Autodesk Fusion 360 part; units mm, degrees
(part 16 of 25)
  arc A4090 (51.0803, 16.2122) -> (51.2018, 15.9188) centre (51.1411, 16.0655) ccw
  arc A4091 (50.459, 16.2243) -> (50.459, 15.9068) centre (50.459, 16.0655) ccw
  arc A4092 (53.8327, 16.4318) -> (54.0572, 16.2072) centre (53.9449, 16.3195) ccw
  arc A4093 (54.9592, 17.78) -> (54.6417, 17.78) centre (54.8005, 17.78) ccw
  arc A4094 (54.9128, 17.0628) -> (54.6882, 17.2873) centre (54.8005, 17.175) ccw
  arc A4095 (49.2443, 18.121) -> (48.9268, 18.121) centre (49.0856, 18.121) ccw
  arc A4096 (49.2343, 18.8634) -> (49.4588, 18.6389) centre (49.3465, 18.7512) ccw
  arc A4097 (53.34, 16.1608) -> (53.34, 16.4783) centre (53.34, 16.3195) ccw
  arc A4098 (52.3619, 16.6927) -> (52.1374, 16.9172) centre (52.2497, 16.805) ccw
  line L1395 (49.3465, 18.7512) -> (49.0855, 18.121)
  arc A4099 (53.34, 17.9387) -> (53.34, 17.6212) centre (53.34, 17.78) ccw
  line L1396 (52.735, 16.3195) -> (53.34, 16.3195)
  arc A4100 (49.8896, 16.4732) -> (49.7681, 16.1798) centre (49.8289, 16.3265) ccw
  arc A4101 (53.1812, 16.3195) -> (53.4987, 16.3195) centre (53.34, 16.3195) ccw
  arc A4102 (51.8319, 16.1798) -> (51.7104, 16.4732) centre (51.7712, 16.3265) ccw
  arc A4103 (53.4988, 17.78) -> (53.1813, 17.78) centre (53.3401, 17.78) ccw
  line L1397 (53.34, 16.3195) -> (53.34, 17.78)
  line L1398 (49.8288, 16.3265) -> (50.459, 16.0655)
  line L1399 (50.459, 16.0655) -> (51.141, 16.0655)
  line L1400 (49.0855, 17.439) -> (49.3465, 16.8088)
  arc A4104 (52.735, 16.4783) -> (52.735, 16.1608) centre (52.735, 16.3195) ccw
  line L1401 (49.0855, 18.121) -> (49.0855, 17.439)
  arc A4105 (50.3982, 15.9188) -> (50.5197, 16.2122) centre (50.459, 16.0655) ccw
  arc A4106 (54.8005, 17.6212) -> (54.8005, 17.9387) centre (54.8005, 17.78) ccw
  arc A4107 (53.34, 17.6212) -> (53.34, 17.9387) centre (53.34, 17.78) ccw
  arc A4108 (49.7166, 16.2143) -> (49.9411, 16.4388) centre (49.8288, 16.3266) ccw
  arc A4109 (49.2322, 17.4997) -> (48.9388, 17.3782) centre (49.0855, 17.439) ccw
  arc A4110 (49.4588, 16.9211) -> (49.2343, 16.6966) centre (49.3465, 16.8089) ccw
  arc A4111 (53.4988, 17.78) -> (53.1813, 17.78) centre (53.3401, 17.78) ccw
  arc A4112 (73.8187, 45.72) -> (73.5012, 45.72) centre (73.66, 45.72) ccw
  line L1402 (49.53, 40.64) -> (50.8, 41.91)
  arc A4113 (13.8113, 33.909) -> (14.1288, 33.909) centre (13.9701, 33.909) ccw
  arc A4114 (21.59, 12.5413) -> (21.59, 12.8588) centre (21.59, 12.7001) ccw
  line L1403 (33.02, 6.35) -> (35.56, 6.35)
  arc A4115 (15.1531, 11.5296) -> (15.3777, 11.305) centre (15.2654, 11.4173) ccw
  arc A4116 (72.5023, 47.1023) -> (72.2777, 46.8777) centre (72.39, 46.99) ccw
  arc A4117 (35.56, 6.1913) -> (35.56, 6.5088) centre (35.56, 6.3501) ccw
  arc A4118 (80.7491, 2.7242) -> (80.7491, 3.0417) centre (80.7491, 2.883) ccw
  arc A4119 (73.8187, 44.45) -> (73.5012, 44.45) centre (73.66, 44.45) ccw
  line L1404 (80.7212, 16.7894) -> (74.2188, 16.7894)
  arc A4120 (16.5481, 12.8588) -> (16.5481, 12.5413) centre (16.5481, 12.7001) ccw
  arc A4121 (3.1603, 40.2443) -> (2.9357, 40.0197) centre (3.048, 40.132) ccw
  line L1405 (80.7491, 2.8829) -> (74.2467, 2.8829)
  line L1406 (21.59, 12.7) -> (22.86, 13.97)
  arc A4122 (13.8577, 35.4477) -> (14.0823, 35.6723) centre (13.97, 35.56) ccw
  line L1407 (3.048, 41.91) -> (3.048, 40.132)
  arc A4123 (14.1288, 35.56) -> (13.8113, 35.56) centre (13.9701, 35.56) ccw
  arc A4124 (72.2313, 46.99) -> (72.5487, 46.99) centre (72.39, 46.99) ccw
  arc A4125 (80.7212, 16.6306) -> (80.7212, 16.9482) centre (80.7212, 16.7894) ccw
  line L1408 (50.8, 41.91) -> (52.07, 43.18)
  arc A4126 (11.43, 37.9413) -> (11.43, 38.2587) centre (11.43, 38.1) ccw
  arc A4127 (43.2923, 40.5277) -> (43.0677, 40.7523) centre (43.18, 40.64) ccw
  arc A4128 (50.6877, 42.0223) -> (50.9123, 41.7977) centre (50.8, 41.91) ccw
  line L1409 (13.97, 35.56) -> (13.97, 33.909)
  arc A4129 (33.02, 6.5088) -> (33.02, 6.1913) centre (33.02, 6.3501) ccw
  arc A4130 (73.5477, 45.6077) -> (73.7723, 45.8323) centre (73.66, 45.72) ccw
  line L1410 (3.048, 40.132) -> (5.08, 38.1)
  arc A4131 (74.2467, 3.0417) -> (74.2467, 2.7242) centre (74.2467, 2.883) ccw
  line L1411 (52.07, 43.18) -> (58.42, 43.18)
  line L1412 (43.18, 40.64) -> (49.53, 40.64)
  arc A4132 (21.4777, 12.8123) -> (21.7023, 12.5877) centre (21.59, 12.7) ccw
  arc A4133 (74.2188, 16.6306) -> (74.2188, 16.9482) centre (74.2188, 16.7894) ccw
  arc A4134 (50.6877, 29.0977) -> (50.9123, 29.3223) centre (50.8, 29.21) ccw
  arc A4135 (5.08, 38.2587) -> (5.08, 37.9413) centre (5.08, 38.1) ccw
  line L1413 (16.5481, 12.7) -> (21.59, 12.7)
  arc A4136 (73.5012, 31.75) -> (73.8187, 31.75) centre (73.66, 31.75) ccw
  arc A4137 (74.2188, 16.9482) -> (74.2188, 16.6306) centre (74.2188, 16.7894) ccw
  arc A4138 (2.8893, 40.132) -> (3.2067, 40.132) centre (3.048, 40.132) ccw
  line L1414 (73.66, 45.72) -> (72.39, 46.99)
  arc A4139 (68.4213, 19.05) -> (68.7387, 19.05) centre (68.58, 19.05) ccw
  arc A4140 (16.6604, 12.5877) -> (16.4358, 12.8123) centre (16.5481, 12.7) ccw
  arc A4141 (50.9588, 29.21) -> (50.6413, 29.21) centre (50.8001, 29.21) ccw
  line L1415 (15.2654, 11.4173) -> (16.5481, 12.7)
  arc A4142 (3.2067, 41.91) -> (2.8893, 41.91) centre (3.048, 41.91) ccw
  arc A4143 (49.53, 40.4813) -> (49.53, 40.7987) centre (49.53, 40.64) ccw
  arc A4144 (40.5277, 38.2123) -> (40.7523, 37.9877) centre (40.64, 38.1) ccw
  line L1416 (22.86, 13.97) -> (22.86, 16.51)
  arc A4145 (43.18, 40.7987) -> (43.18, 40.4813) centre (43.18, 40.64) ccw
  arc A4146 (22.7012, 13.97) -> (23.0188, 13.97) centre (22.86, 13.97) ccw
  line L1417 (40.64, 33.02) -> (46.99, 33.02)
  arc A4147 (47.1023, 33.1323) -> (46.8777, 32.9077) centre (46.99, 33.02) ccw
  line L1418 (73.66, 44.45) -> (73.66, 45.72)
  line L1419 (5.08, 38.1) -> (11.43, 38.1)
  line L1420 (73.66, 31.75) -> (73.66, 44.45)
  arc A4148 (11.5423, 38.2123) -> (11.3177, 37.9877) centre (11.43, 38.1) ccw
  line L1421 (11.43, 38.1) -> (13.97, 35.56)
  line L1422 (72.39, 46.99) -> (72.39, 49.53)
  arc A4149 (4.9677, 37.9877) -> (5.1923, 38.2123) centre (5.08, 38.1) ccw
  arc A4150 (23.0188, 16.51) -> (22.7012, 16.51) centre (22.86, 16.51) ccw
  arc A4151 (22.9723, 13.8577) -> (22.7477, 14.0823) centre (22.86, 13.97) ccw
  arc A4152 (73.5012, 44.45) -> (73.8187, 44.45) centre (73.66, 44.45) ccw
  arc A4153 (72.5487, 49.53) -> (72.2313, 49.53) centre (72.39, 49.53) ccw
  arc A4154 (16.002, 26.0668) -> (16.002, 25.7492) centre (16.002, 25.908) ccw
  arc A4155 (73.5012, 29.21) -> (73.8187, 29.21) centre (73.66, 29.21) ccw
  line L1423 (63.5, 31.75) -> (63.5, 29.21)
  arc A4156 (40.64, 33.1788) -> (40.64, 32.8613) centre (40.64, 33.0201) ccw
  line L1424 (68.58, 20.32) -> (70.485, 22.225)
  arc A4157 (26.5113, 25.4) -> (26.8288, 25.4) centre (26.67, 25.4) ccw
  line L1425 (68.58, 19.05) -> (68.58, 20.32)
  line L1426 (26.67, 29.21) -> (26.67, 25.4)
  arc A4158 (58.42, 43.0213) -> (58.42, 43.3387) centre (58.42, 43.18) ccw
  line L1427 (46.99, 33.02) -> (50.8, 29.21)
  line L1428 (33.02, 6.35) -> (30.48, 6.35)
  arc A4159 (26.67, 25.2413) -> (26.67, 25.5588) centre (26.67, 25.4001) ccw
  arc A4160 (73.7723, 29.0977) -> (73.5477, 29.3223) centre (73.66, 29.21) ccw
  line L1429 (73.66, 29.21) -> (73.66, 31.75)
  line L1430 (50.8, 29.21) -> (50.8, 25.4)
  arc A4161 (30.3677, 6.2377) -> (30.5923, 6.4623) centre (30.48, 6.35) ccw
  arc A4162 (46.99, 32.8613) -> (46.99, 33.1788) centre (46.99, 33.0201) ccw
  line L1431 (72.39, 27.94) -> (70.485, 27.94)
  arc A4163 (68.4677, 20.4323) -> (68.6923, 20.2077) centre (68.58, 20.32) ccw
  line L1432 (73.66, 29.21) -> (72.39, 27.94)
  arc A4164 (21.59, 25.5588) -> (21.59, 25.2413) centre (21.59, 25.4001) ccw
  arc A4165 (52.07, 43.3387) -> (52.07, 43.0213) centre (52.07, 43.18) ccw
  arc A4166 (49.4177, 40.7523) -> (49.6423, 40.5277) centre (49.53, 40.64) ccw
  arc A4167 (21.1943, 26.0203) -> (20.9697, 25.7957) centre (21.082, 25.908) ccw
  arc A4168 (70.8406, 16.9482) -> (70.8406, 16.6306) centre (70.8406, 16.7894) ccw
  arc A4169 (37.9877, 30.5923) -> (38.2123, 30.3677) centre (38.1, 30.48) ccw
  arc A4170 (22.9723, 14.0823) -> (22.7477, 13.8577) centre (22.86, 13.97) ccw
  arc A4171 (21.4777, 25.2877) -> (21.7023, 25.5123) centre (21.59, 25.4) ccw
  arc A4172 (50.6413, 25.4) -> (50.9588, 25.4) centre (50.8001, 25.4) ccw
  line L1433 (16.002, 25.908) -> (21.082, 25.908)
  arc A4173 (63.6587, 31.75) -> (63.3413, 31.75) centre (63.5, 31.75) ccw
  arc A4174 (70.7283, 16.6771) -> (70.9529, 16.9017) centre (70.8406, 16.7894) ccw
  line L1434 (70.485, 22.225) -> (70.485, 27.94)
  line L1435 (40.64, 33.02) -> (38.1, 30.48)
  arc A4175 (63.3413, 29.21) -> (63.6587, 29.21) centre (63.5, 29.21) ccw
  arc A4176 (33.02, 6.1913) -> (33.02, 6.5088) centre (33.02, 6.3501) ccw
  arc A4177 (64.77, 28.0988) -> (64.77, 27.7813) centre (64.77, 27.9401) ccw
  arc A4178 (70.485, 28.0988) -> (70.485, 27.7813) centre (70.485, 27.9401) ccw
  arc A4179 (68.7387, 20.32) -> (68.4213, 20.32) centre (68.58, 20.32) ccw
  arc A4180 (70.3263, 22.225) -> (70.6437, 22.225) centre (70.485, 22.225) ccw
  arc A4181 (70.5973, 22.1127) -> (70.3727, 22.3373) centre (70.485, 22.225) ccw
  arc A4182 (26.5577, 29.3223) -> (26.7823, 29.0977) centre (26.67, 29.21) ccw
  arc A4183 (21.082, 25.7492) -> (21.082, 26.0668) centre (21.082, 25.908) ccw
  line L1436 (74.2188, 16.7894) -> (70.8406, 16.7894)
  arc A4184 (28.0523, 30.3677) -> (27.8277, 30.5923) centre (27.94, 30.48) ccw
  arc A4185 (70.6437, 27.94) -> (70.3263, 27.94) centre (70.485, 27.94) ccw
  arc A4186 (73.8187, 31.75) -> (73.5012, 31.75) centre (73.66, 31.75) ccw
  line L1437 (70.8406, 16.7894) -> (68.58, 19.05)
  arc A4187 (50.9123, 41.7977) -> (50.6877, 42.0223) centre (50.8, 41.91) ccw
  arc A4188 (27.94, 30.6388) -> (27.94, 30.3212) centre (27.94, 30.48) ccw
  line L1438 (30.48, 6.35) -> (22.86, 13.97)
  line L1439 (64.77, 27.94) -> (70.485, 27.94)
  arc A4189 (30.48, 6.5088) -> (30.48, 6.1913) centre (30.48, 6.3501) ccw
  arc A4190 (72.2777, 28.0523) -> (72.5023, 27.8277) centre (72.39, 27.94) ccw
  line L1440 (21.59, 25.4) -> (26.67, 25.4)
  arc A4191 (40.7523, 32.9077) -> (40.5277, 33.1323) centre (40.64, 33.02) ccw
  arc A4192 (52.1823, 43.0677) -> (51.9577, 43.2923) centre (52.07, 43.18) ccw
  line L1441 (21.082, 25.908) -> (21.59, 25.4)
  line L1442 (38.1, 30.48) -> (27.94, 30.48)
  line L1443 (40.64, 38.1) -> (43.18, 40.64)
  line L1444 (63.5, 29.21) -> (64.77, 27.94)
  arc A4193 (68.6923, 19.1623) -> (68.4677, 18.9377) centre (68.58, 19.05) ccw
  arc A4194 (71.12, 39.2938) -> (71.12, 39.4462) centre (71.12, 39.37) ccw
  arc A4195 (52.1239, 39.3161) -> (52.0161, 39.4239) centre (52.07, 39.37) ccw
  arc A4196 (16.8402, 44.196) -> (16.6878, 44.196) centre (16.764, 44.196) ccw
  line L1445 (13.081, 30.48) -> (9.271, 34.29)
  arc A4197 (3.048, 34.3662) -> (3.048, 34.2138) centre (3.048, 34.29) ccw
  line L1446 (78.74, 31.75) -> (78.74, 44.45)
  arc A4198 (14.0239, 47.0439) -> (13.9161, 46.9361) centre (13.97, 46.99) ccw
  arc A4199 (8.128, 34.2138) -> (8.128, 34.3662) centre (8.128, 34.29) ccw
  arc A4200 (13.8938, 46.99) -> (14.0462, 46.99) centre (13.97, 46.99) ccw
  line L1447 (54.61, 36.83) -> (71.12, 36.83)
  arc A4201 (45.7962, 13.97) -> (45.6438, 13.97) centre (45.72, 13.97) ccw
  arc A4202 (50.7461, 33.0739) -> (50.8539, 32.9661) centre (50.8, 33.02) ccw
  line L1448 (52.07, 39.37) -> (71.12, 39.37)
  arc A4203 (76.1238, 31.75) -> (76.2762, 31.75) centre (76.2, 31.75) ccw
  arc A4204 (64.6577, 27.8277) -> (64.8823, 28.0523) centre (64.77, 27.94) ccw
  arc A4205 (52.07, 39.4462) -> (52.07, 39.2938) centre (52.07, 39.37) ccw
  arc A4206 (54.61, 36.9062) -> (54.61, 36.7538) centre (54.61, 36.83) ccw
  arc A4207 (72.39, 27.7813) -> (72.39, 28.0988) centre (72.39, 27.9401) ccw
  line L1449 (50.8, 33.02) -> (54.61, 36.83)
  arc A4208 (14.0462, 49.53) -> (13.8938, 49.53) centre (13.97, 49.53) ccw
  line L1450 (45.72, 13.97) -> (45.72, 6.35)
  line L1451 (16.764, 44.196) -> (16.764, 32.004)
  arc A4209 (54.6639, 36.7761) -> (54.5561, 36.8839) centre (54.61, 36.83) ccw
  arc A4210 (78.6638, 31.75) -> (78.8162, 31.75) centre (78.74, 31.75) ccw
  line L1452 (16.764, 32.004) -> (15.24, 30.48)
  arc A4211 (16.6878, 32.004) -> (16.8402, 32.004) centre (16.764, 32.004) ccw
  arc A4212 (13.0271, 30.4261) -> (13.1349, 30.5339) centre (13.081, 30.48) ccw
  arc A4213 (8.128, 34.3662) -> (8.128, 34.2138) centre (8.128, 34.29) ccw
  arc A4214 (11.3538, 45.72) -> (11.5062, 45.72) centre (11.43, 45.72) ccw
  line L1453 (27.94, 30.48) -> (26.67, 29.21)
  arc A4215 (78.8162, 44.45) -> (78.6638, 44.45) centre (78.74, 44.45) ccw
  arc A4216 (63.6123, 29.3223) -> (63.3877, 29.0977) centre (63.5, 29.21) ccw
  arc A4217 (70.485, 27.7813) -> (70.485, 28.0988) centre (70.485, 27.9401) ccw
  arc A4218 (16.7101, 44.1421) -> (16.8179, 44.2499) centre (16.764, 44.196) ccw
  arc A4219 (74.2467, 7.4803) -> (74.2467, 7.3279) centre (74.2467, 7.4041) ccw
  line L1454 (80.7491, 7.4041) -> (82.677, 9.332)
  line L1455 (13.97, 46.99) -> (16.764, 44.196)
  arc A4220 (10.1061, 44.5039) -> (10.2139, 44.3961) centre (10.16, 44.45) ccw
  arc A4221 (76.2762, 44.45) -> (76.1238, 44.45) centre (76.2, 44.45) ccw
  arc A4222 (55.8038, 19.05) -> (55.9562, 19.05) centre (55.88, 19.05) ccw
  arc A4223 (13.081, 30.5562) -> (13.081, 30.4038) centre (13.081, 30.48) ccw
  arc A4224 (55.9339, 19.1039) -> (55.8261, 18.9961) centre (55.88, 19.05) ccw
  arc A4225 (80.6953, 7.458) -> (80.803, 7.3502) centre (80.7492, 7.4041) ccw
  arc A4226 (38.1, 30.3212) -> (38.1, 30.6388) centre (38.1, 30.48) ccw
  arc A4227 (50.7461, 38.1539) -> (50.8539, 38.0461) centre (50.8, 38.1) ccw
  line L1456 (3.048, 34.29) -> (8.128, 34.29)
  line L1457 (50.8, 38.1) -> (52.07, 39.37)
  arc A4228 (9.271, 34.2138) -> (9.271, 34.3662) centre (9.271, 34.29) ccw
  arc A4229 (26.8288, 29.21) -> (26.5113, 29.21) centre (26.67, 29.21) ccw
  arc A4230 (45.6438, 6.35) -> (45.7962, 6.35) centre (45.72, 6.35) ccw
  line L1458 (9.271, 34.29) -> (8.128, 34.29)
  line L1459 (76.2, 31.75) -> (76.2, 44.45)
  arc A4231 (16.8179, 31.9501) -> (16.7101, 32.0579) centre (16.764, 32.004) ccw
  arc A4232 (71.12, 36.7538) -> (71.12, 36.9062) centre (71.12, 36.83) ccw
  line L1460 (15.24, 30.48) -> (13.081, 30.48)
  arc A4233 (15.1861, 30.5339) -> (15.2939, 30.4261) centre (15.24, 30.48) ccw
  arc A4234 (15.24, 30.4038) -> (15.24, 30.5562) centre (15.24, 30.48) ccw
  line L1461 (13.97, 49.53) -> (13.97, 46.99)
  arc A4235 (9.3249, 34.3439) -> (9.2171, 34.2361) centre (9.271, 34.29) ccw
  line L1462 (71.7067, 7.4041) -> (68.9508, 10.16)
  arc A4236 (11.5062, 49.53) -> (11.3538, 49.53) centre (11.43, 49.53) ccw
  arc A4237 (33.02, 44.5262) -> (33.02, 44.3738) centre (33.02, 44.45) ccw
  arc A4238 (60.9061, 45.6661) -> (61.0139, 45.7739) centre (60.96, 45.72) ccw
  line L1463 (40.64, 41.91) -> (43.18, 44.45)
  arc A4239 (39.3161, 44.5039) -> (39.4239, 44.3961) centre (39.37, 44.45) ccw
  line L1464 (60.96, 45.72) -> (59.69, 46.99)
  arc A4240 (69.0047, 10.2139) -> (68.897, 10.1061) centre (68.9509, 10.16) ccw
  line L1465 (58.42, 16.51) -> (67.31, 16.51)
  line L1466 (11.43, 45.72) -> (11.43, 49.53)
  arc A4241 (61.0362, 45.72) -> (60.8838, 45.72) centre (60.96, 45.72) ccw
  arc A4242 (82.7532, 12.446) -> (82.6008, 12.446) centre (82.677, 12.446) ccw
  arc A4243 (82.7309, 9.2781) -> (82.6231, 9.3858) centre (82.677, 9.332) ccw
  arc A4244 (71.6529, 7.3502) -> (71.7606, 7.458) centre (71.7067, 7.4041) ccw
  line L1467 (55.88, 34.29) -> (55.88, 19.05)
  arc A4245 (58.42, 16.5862) -> (58.42, 16.4338) centre (58.42, 16.51) ccw
  line L1468 (43.18, 48.26) -> (44.45, 46.99)
  line L1469 (59.69, 46.99) -> (44.45, 46.99)
  arc A4246 (8.128, 44.5262) -> (8.128, 44.3738) centre (8.128, 44.45) ccw
  arc A4247 (36.7761, 38.1539) -> (36.8839, 38.0461) centre (36.83, 38.1) ccw
  arc A4248 (11.4839, 45.6661) -> (11.3761, 45.7739) centre (11.43, 45.72) ccw
  arc A4249 (30.4261, 41.9639) -> (30.5339, 41.8561) centre (30.48, 41.91) ccw
  line L1470 (60.96, 43.18) -> (60.96, 45.72)
  line L1471 (10.16, 44.45) -> (11.43, 45.72)
  arc A4250 (55.9562, 34.29) -> (55.8038, 34.29) centre (55.88, 34.29) ccw
  arc A4251 (71.7067, 7.4803) -> (71.7067, 7.3279) centre (71.7067, 7.4041) ccw
  arc A4252 (34.29, 38.1762) -> (34.29, 38.0238) centre (34.29, 38.1) ccw
  line L1472 (39.37, 44.45) -> (33.02, 44.45)
  arc A4253 (59.7439, 47.0439) -> (59.6361, 46.9361) centre (59.69, 46.99) ccw
  arc A4254 (43.18, 44.5262) -> (43.18, 44.3738) centre (43.18, 44.45) ccw
  arc A4255 (43.2339, 48.3139) -> (43.1261, 48.2061) centre (43.18, 48.26) ccw
  line L1473 (43.18, 48.26) -> (39.37, 44.45)
  line L1474 (30.48, 35.56) -> (31.75, 34.29)
  arc A4256 (53.34, 44.3738) -> (53.34, 44.5262) centre (53.34, 44.45) ccw
  arc A4257 (40.6939, 41.8561) -> (40.5861, 41.9639) centre (40.64, 41.91) ccw
  arc A4258 (59.69, 46.9138) -> (59.69, 47.0662) centre (59.69, 46.99) ccw
  line L1475 (55.88, 19.05) -> (58.42, 16.51)
  arc A4259 (40.5861, 41.9639) -> (40.6939, 41.8561) centre (40.64, 41.91) ccw
  line L1476 (31.75, 34.29) -> (34.29, 34.29)
  arc A4260 (82.6008, 9.332) -> (82.7532, 9.332) centre (82.677, 9.332) ccw
  line L1477 (71.7067, 7.4041) -> (74.2467, 7.4041)
  arc A4261 (74.2467, 7.3279) -> (74.2467, 7.4803) centre (74.2467, 7.4041) ccw
  line L1478 (82.677, 9.332) -> (82.677, 12.446)
  arc A4262 (43.2562, 49.53) -> (43.1038, 49.53) centre (43.18, 49.53) ccw
  line L1479 (33.02, 44.45) -> (30.48, 41.91)
  line L1480 (36.83, 38.1) -> (40.64, 41.91)
  line L1481 (8.128, 44.45) -> (10.16, 44.45)
  arc A4263 (43.2339, 48.2061) -> (43.1261, 48.3139) centre (43.18, 48.26) ccw
  line L1482 (80.7491, 7.4041) -> (74.2467, 7.4041)
  arc A4264 (60.8838, 43.18) -> (61.0362, 43.18) centre (60.96, 43.18) ccw
  arc A4265 (44.3961, 46.9361) -> (44.5039, 47.0439) centre (44.45, 46.99) ccw
  arc A4266 (33.0739, 44.3961) -> (32.9661, 44.5039) centre (33.02, 44.45) ccw
  arc A4267 (10.16, 44.3738) -> (10.16, 44.5262) centre (10.16, 44.45) ccw
  line L1483 (67.31, 10.16) -> (68.9508, 10.16)
  arc A4268 (67.31, 16.4338) -> (67.31, 16.5862) centre (67.31, 16.51) ccw
  arc A4269 (80.7491, 7.3279) -> (80.7491, 7.4803) centre (80.7491, 7.4041) ccw
  line L1484 (43.18, 49.53) -> (43.18, 48.26)
  arc A4270 (43.1038, 48.26) -> (43.2562, 48.26) centre (43.18, 48.26) ccw
  arc A4271 (43.2339, 44.3961) -> (43.1261, 44.5039) centre (43.18, 44.45) ccw
  arc A4272 (30.5339, 35.6139) -> (30.4261, 35.5061) centre (30.48, 35.56) ccw
  arc A4273 (68.9508, 10.0838) -> (68.9508, 10.2362) centre (68.9508, 10.16) ccw
  arc A4274 (58.3661, 16.4561) -> (58.4739, 16.5639) centre (58.42, 16.51) ccw
  arc A4275 (67.31, 10.2362) -> (67.31, 10.0838) centre (67.31, 10.16) ccw
  arc A4276 (34.29, 34.2138) -> (34.29, 34.3662) centre (34.29, 34.29) ccw
  line L1485 (35.56, 46.99) -> (34.29, 45.72)
  line L1486 (34.29, 38.1) -> (36.83, 38.1)
  arc A4277 (77.2956, 53.9596) -> (77.5596, 53.7832) centre (77.4276, 53.8714) ccw
  arc A4278 (44.45, 47.0662) -> (44.45, 46.9138) centre (44.45, 46.99) ccw
  line L1487 (43.18, 44.45) -> (53.34, 44.45)
  arc A4279 (31.6961, 34.2361) -> (31.8039, 34.3439) centre (31.75, 34.29) ccw
  line L1488 (30.48, 41.91) -> (30.48, 35.56)
  arc A4280 (45.72, 25.4762) -> (45.72, 25.3238) centre (45.72, 25.4) ccw
  arc A4281 (46.2739, 21.7523) -> (46.2739, 22.0698) centre (46.2739, 21.9111) ccw
  arc A4282 (24.765, 45.7962) -> (24.765, 45.6438) centre (24.765, 45.72) ccw
  line L1489 (40.64, 6.35) -> (39.1287, 6.35)
  arc A4283 (35.6139, 46.9361) -> (35.5061, 47.0439) centre (35.56, 46.99) ccw
  arc A4284 (7.6739, 29.2639) -> (7.5661, 29.1561) centre (7.62, 29.21) ccw
  line L1490 (34.29, 45.72) -> (24.765, 45.72)
  arc A4285 (48.26, 25.3238) -> (48.26, 25.4762) centre (48.26, 25.4) ccw
  arc A4286 (29.4513, 49.6888) -> (29.4513, 49.3713) centre (29.4513, 49.5301) ccw
  arc A4287 (39.1287, 6.5087) -> (39.1287, 6.1912) centre (39.1287, 6.35) ccw
  arc A4288 (24.8189, 29.1561) -> (24.7111, 29.2639) centre (24.765, 29.21) ccw
  arc A4289 (35.4838, 46.99) -> (35.6362, 46.99) centre (35.56, 46.99) ccw
  line L1491 (45.72, 25.4) -> (40.64, 30.48)
  arc A4290 (38.1, 6.5088) -> (38.1, 6.1913) centre (38.1, 6.3501) ccw
  arc A4291 (30.3212, 49.53) -> (30.6387, 49.53) centre (30.48, 49.53) ccw
  arc A4292 (39.37, 44.3738) -> (39.37, 44.5262) centre (39.37, 44.45) ccw
  arc A4293 (40.6939, 30.5339) -> (40.5861, 30.4261) centre (40.64, 30.48) ccw
  line L1492 (29.4513, 49.53) -> (30.48, 49.53)
  arc A4294 (30.48, 49.3713) -> (30.48, 49.6888) centre (30.48, 49.5301) ccw
  arc A4295 (38.1, 6.5087) -> (38.1, 6.1912) centre (38.1, 6.35) ccw
  arc A4296 (40.7987, 6.35) -> (40.4812, 6.35) centre (40.6399, 6.35) ccw
  arc A4297 (53.34, 19.3992) -> (53.34, 19.0817) centre (53.34, 19.2405) ccw
  arc A4298 (39.1287, 6.1912) -> (39.1287, 6.5087) centre (39.1287, 6.35) ccw
  arc A4299 (54.6882, 18.2727) -> (54.9128, 18.4972) centre (54.8005, 18.385) ccw
  arc A4300 (40.64, 6.1912) -> (40.64, 6.5087) centre (40.64, 6.35) ccw
  arc A4301 (8.8361, 27.8861) -> (8.9439, 27.9939) centre (8.89, 27.94) ccw
  line L1493 (23.495, 27.94) -> (24.765, 29.21)
  arc A4302 (45.6661, 25.3461) -> (45.7739, 25.4539) centre (45.72, 25.4) ccw
  line L1494 (48.26, 25.4) -> (45.72, 25.4)
  arc A4303 (34.29, 45.6438) -> (34.29, 45.7962) centre (34.29, 45.72) ccw
  arc A4304 (31.75, 34.3662) -> (31.75, 34.2138) centre (31.75, 34.29) ccw
  arc A4305 (40.4812, 6.35) -> (40.7987, 6.35) centre (40.6399, 6.35) ccw
  line L1495 (38.1, 6.35) -> (40.64, 6.35)
  arc A4306 (34.2361, 45.7739) -> (34.3439, 45.6661) centre (34.29, 45.72) ccw
  line L1496 (30.48, 49.53) -> (27.94, 49.53)
  arc A4307 (23.4411, 27.9939) -> (23.5489, 27.8861) centre (23.495, 27.94) ccw
  arc A4308 (76.9116, 52.4192) -> (76.9116, 52.1017) centre (76.9116, 52.2604) ccw
  line L1497 (76.9346, 51.3926) -> (77.0064, 51.0316)
  line L1498 (39.1287, 6.35) -> (38.1, 6.35)
  arc A4309 (8.89, 28.0162) -> (8.89, 27.8638) centre (8.89, 27.94) ccw
  arc A4310 (37.9413, 6.35) -> (38.2588, 6.35) centre (38.1, 6.35) ccw
  line L1499 (7.62, 29.21) -> (8.89, 27.94)
  arc A4311 (30.4038, 35.56) -> (30.5562, 35.56) centre (30.48, 35.56) ccw
  arc A4312 (30.5562, 41.91) -> (30.4038, 41.91) centre (30.48, 41.91) ccw
  arc A4313 (35.6362, 49.53) -> (35.4838, 49.53) centre (35.56, 49.53) ccw
  line L1500 (23.495, 27.94) -> (8.89, 27.94)
  arc A4314 (23.495, 27.8638) -> (23.495, 28.0162) centre (23.495, 27.94) ccw
  line L1501 (35.56, 46.99) -> (35.56, 49.53)
  arc A4315 (38.2588, 6.35) -> (37.9413, 6.35) centre (38.1, 6.35) ccw
  line L1502 (80.3275, 52.2605) -> (80.3275, 51.6255)
  line L1503 (77.8657, 54.462) -> (77.6322, 54.1775)
  arc A4316 (36.83, 38.0238) -> (36.83, 38.1762) centre (36.83, 38.1) ccw
  arc A4317 (40.64, 6.1913) -> (40.64, 6.5088) centre (40.64, 6.3501) ccw
  arc A4318 (30.6387, 49.53) -> (30.3212, 49.53) centre (30.48, 49.53) ccw
  arc A4319 (79.5941, 55.3734) -> (79.5019, 55.6772) centre (79.548, 55.5253) ccw
  arc A4320 (78.2382, 54.6101) -> (78.0137, 54.8346) centre (78.126, 54.7224) ccw
  line L1504 (77.0064, 51.0316) -> (77.1133, 50.6793)
  arc A4321 (76.9613, 50.6332) -> (77.2652, 50.7254) centre (77.1133, 50.6793) ccw
  line L1505 (76.9116, 52.2605) -> (80.3275, 52.2605)
  arc A4322 (77.1621, 52.8235) -> (76.8507, 52.8854) centre (77.0064, 52.8545) ccw
  arc A4323 (27.94, 49.6888) -> (27.94, 49.3713) centre (27.94, 49.5301) ccw
  arc A4324 (79.4421, 55.3281) -> (79.3206, 55.6214) centre (79.3813, 55.4748) ccw
  line L1506 (77.6322, 54.1775) -> (77.4276, 53.8714)
  arc A4325 (78.8048, 55.0284) -> (78.6284, 55.2923) centre (78.7166, 55.1604) ccw
  arc A4326 (77.1583, 51.0777) -> (76.8545, 50.9855) centre (77.0064, 51.0316) ccw
  arc A4327 (79.1161, 55.1939) -> (78.9664, 55.4739) centre (79.0413, 55.3339) ccw
  arc A4328 (77.0926, 52.4778) -> (76.7766, 52.5089) centre (76.9346, 52.4934) ccw
  line L1507 (78.4105, 54.9558) -> (78.126, 54.7223)
  line L1508 (79.0412, 55.3339) -> (78.7166, 55.1604)
  line L1509 (79.3813, 55.4747) -> (79.0412, 55.3339)
  arc A4329 (79.3352, 55.6267) -> (79.4274, 55.3228) centre (79.3813, 55.4747) ccw
  line L1510 (78.126, 54.7223) -> (77.8657, 54.462)
  arc A4330 (76.8507, 51.0006) -> (77.1621, 51.0625) centre (77.0064, 51.0316) ccw
  arc A4331 (77.0903, 51.4236) -> (76.7789, 51.3616) centre (76.9346, 51.3926) ccw
  arc A4332 (78.9805, 55.4805) -> (79.102, 55.1872) centre (79.0413, 55.3338) ccw
  arc A4333 (27.94, 49.6887) -> (27.94, 49.3712) centre (27.94, 49.53) ccw
  arc A4334 (78.6418, 55.3004) -> (78.7914, 55.0203) centre (78.7166, 55.1604) ccw
  arc A4335 (82.1739, 48.6921) -> (82.3236, 48.4121) centre (82.2488, 48.5521) ccw
  arc A4336 (80.4862, 51.6255) -> (80.1688, 51.6255) centre (80.3275, 51.6255) ccw
  arc A4337 (77.0696, 51.6411) -> (76.7537, 51.6099) centre (76.9116, 51.6255) ccw
  line L1511 (77.1133, 53.2067) -> (77.0064, 52.8544)
  arc A4338 (77.5676, 53.7966) -> (77.2876, 53.9462) centre (77.4276, 53.8714) ccw
  arc A4339 (77.9884, 54.3613) -> (77.743, 54.5627) centre (77.8657, 54.462) ccw
  line L1512 (76.9346, 52.4934) -> (76.9116, 52.2605)
  arc A4340 (82.3095, 48.4055) -> (82.188, 48.6988) centre (82.2487, 48.5522) ccw
  line L1513 (78.7166, 55.1604) -> (78.4105, 54.9558)
  arc A4341 (80.3275, 52.1017) -> (80.3275, 52.4192) centre (80.3275, 52.2604) ccw
  arc A4342 (76.7766, 51.377) -> (77.0926, 51.4082) centre (76.9346, 51.3926) ccw
  arc A4343 (77.1141, 53.6216) -> (77.3941, 53.4719) centre (77.2541, 53.5468) ccw
  arc A4344 (78.3223, 55.0878) -> (78.4987, 54.8238) centre (78.4105, 54.9558) ccw
  arc A4345 (80.1687, 51.6255) -> (80.4862, 51.6255) centre (80.3274, 51.6255) ccw
  arc A4346 (28.0988, 49.53) -> (27.7813, 49.53) centre (27.9401, 49.53) ccw
  line L1514 (77.2541, 53.5468) -> (77.1133, 53.2067)
  arc A4347 (77.7641, 54.0893) -> (77.5002, 54.2657) centre (77.6322, 54.1775) ccw
  arc A4348 (78.5112, 54.8331) -> (78.3098, 55.0786) centre (78.4105, 54.9558) ccw
  arc A4349 (76.8545, 52.9005) -> (77.1583, 52.8083) centre (77.0064, 52.8544) ccw
  arc A4350 (77.2652, 53.1606) -> (76.9613, 53.2528) centre (77.1132, 53.2067) ccw
  line L1515 (76.9116, 51.6255) -> (76.9346, 51.3926)
  line L1516 (79.548, 55.5253) -> (79.3813, 55.4747)
  arc A4351 (76.9116, 51.7843) -> (76.9116, 51.4668) centre (76.9116, 51.6256) ccw
  arc A4352 (78.0253, 54.845) -> (78.2267, 54.5996) centre (78.126, 54.7223) ccw
  arc A4353 (76.7537, 52.2761) -> (77.0696, 52.2449) centre (76.9116, 52.2605) ccw
  arc A4354 (80.3275, 51.4668) -> (80.3275, 51.7843) centre (80.3275, 51.6256) ccw
  arc A4355 (77.4008, 53.486) -> (77.1075, 53.6075) centre (77.2542, 53.5468) ccw
  arc A4356 (77.7534, 54.5743) -> (77.9779, 54.3498) centre (77.8657, 54.4621) ccw
  arc A4357 (30.48, 49.3712) -> (30.48, 49.6887) centre (30.48, 49.53) ccw
  arc A4358 (29.4513, 49.3713) -> (29.4513, 49.6888) centre (29.4513, 49.5301) ccw
  arc A4359 (76.9666, 53.2674) -> (77.2599, 53.1459) centre (77.1132, 53.2066) ccw
  arc A4360 (76.7789, 52.5244) -> (77.0903, 52.4624) centre (76.9346, 52.4934) ccw
  line L1517 (77.4276, 53.8714) -> (77.2541, 53.5468)
  arc A4361 (27.7813, 49.53) -> (28.0988, 49.53) centre (27.9401, 49.53) ccw
  arc A4362 (80.4862, 52.2605) -> (80.1687, 52.2605) centre (80.3274, 52.2605) ccw
  line L1518 (77.0064, 52.8544) -> (76.9346, 52.4934)
  line L1519 (80.3275, 51.6255) -> (76.9116, 51.6255)
  arc A4363 (77.5094, 54.2782) -> (77.7549, 54.0768) centre (77.6322, 54.1775) ccw
  line L1520 (27.94, 49.53) -> (29.4513, 49.53)
  line L1521 (78.126, 49.1637) -> (78.4105, 48.9302)
  arc A4364 (79.102, 48.6988) -> (78.9805, 48.4055) centre (79.0413, 48.5522) ccw
  arc A4365 (80.1688, 48.2096) -> (80.4862, 48.2096) centre (80.3275, 48.2096) ccw
  line L1522 (80.9625, 51.6255) -> (80.9625, 48.2096)
  arc A4366 (78.9664, 48.4121) -> (79.1161, 48.6921) centre (79.0413, 48.5521) ccw
  arc A4367 (77.5002, 49.6203) -> (77.7641, 49.7967) centre (77.6322, 49.7085) ccw
  arc A4368 (80.9469, 48.3676) -> (80.9781, 48.0517) centre (80.9625, 48.2097) ccw
  line L1523 (77.4276, 50.0146) -> (77.6322, 49.7085)
  arc A4369 (80.1102, 48.3906) -> (80.079, 48.0746) centre (80.0946, 48.2326) ccw
  arc A4370 (78.2267, 49.2864) -> (78.0253, 49.041) centre (78.126, 49.1637) ccw
  arc A4371 (81.2109, 48.0746) -> (81.1798, 48.3906) centre (81.1954, 48.2326) ccw
  arc A4372 (82.4852, 48.8576) -> (82.6616, 48.5936) centre (82.5734, 48.7256) ccw
  line L1524 (80.9625, 48.2096) -> (81.1954, 48.2326)
  line L1525 (81.9087, 48.4113) -> (82.2488, 48.5521)
  arc A4373 (77.2599, 50.7401) -> (76.9666, 50.6186) centre (77.1133, 50.6793) ccw
  line L1526 (77.6322, 49.7085) -> (77.8657, 49.424)
  line L1527 (77.2541, 50.3392) -> (77.4276, 50.0146)
  arc A4374 (77.743, 49.3233) -> (77.9884, 49.5247) centre (77.8657, 49.424) ccw
  arc A4375 (81.5874, 48.1487) -> (81.5255, 48.4601) centre (81.5564, 48.3044) ccw
  line L1528 (77.1133, 50.6793) -> (77.2541, 50.3392)
  arc A4376 (78.6284, 48.5936) -> (78.8048, 48.8576) centre (78.7166, 48.7256) ccw
  arc A4377 (78.3098, 48.8074) -> (78.5112, 49.0529) centre (78.4105, 48.9301) ccw
  arc A4378 (79.6875, 48.1525) -> (79.7797, 48.4563) centre (79.7336, 48.3044) ccw
  arc A4379 (79.7645, 48.4601) -> (79.7026, 48.1487) centre (79.7335, 48.3044) ccw
  arc A4380 (81.1212, 51.6255) -> (80.8037, 51.6255) centre (80.9624, 51.6255) ccw
  arc A4381 (80.0636, 48.0769) -> (80.1256, 48.3883) centre (80.0946, 48.2326) ccw
  arc A4382 (78.7914, 48.8656) -> (78.6418, 48.5856) centre (78.7166, 48.7256) ccw
  arc A4383 (81.1644, 48.3883) -> (81.2264, 48.0769) centre (81.1954, 48.2326) ccw
  line L1529 (79.3813, 48.4113) -> (79.7336, 48.3044)
  arc A4384 (78.0137, 49.0514) -> (78.2382, 49.2759) centre (78.126, 49.1637) ccw
  line L1530 (80.3275, 51.6255) -> (80.9625, 51.6255)
  line L1531 (78.7166, 48.7256) -> (79.0412, 48.5521)
  arc A4385 (78.4987, 49.0621) -> (78.3223, 48.7982) centre (78.4105, 48.9302) ccw
  arc A4386 (82.6482, 48.5856) -> (82.4986, 48.8656) centre (82.5734, 48.7256) ccw
  line L1532 (81.1954, 48.2326) -> (81.5564, 48.3044)
  arc A4387 (77.9779, 49.5362) -> (77.7534, 49.3117) centre (77.8657, 49.424) ccw
  arc A4388 (81.5103, 48.4563) -> (81.6025, 48.1525) centre (81.5564, 48.3044) ccw
  arc A4389 (80.8037, 48.2096) -> (81.1212, 48.2096) centre (80.9624, 48.2096) ccw
  arc A4390 (77.3941, 50.4141) -> (77.1141, 50.2644) centre (77.2541, 50.3392) ccw
  arc A4391 (80.9625, 51.4667) -> (80.9625, 51.7842) centre (80.9625, 51.6255) ccw
  line L1533 (77.8657, 49.424) -> (78.126, 49.1637)
  line L1534 (79.0412, 48.5521) -> (79.3813, 48.4113)
  line L1535 (79.7336, 48.3044) -> (80.0946, 48.2326)
  arc A4392 (82.9677, 48.7982) -> (82.7913, 49.0621) centre (82.8795, 48.9301) ccw
  arc A4393 (81.8479, 48.5579) -> (81.9694, 48.2646) centre (81.9086, 48.4113) ccw
  line L1536 (82.2488, 48.5521) -> (82.5734, 48.7256)
  line L1537 (81.5564, 48.3044) -> (81.9087, 48.4113)
  line L1538 (82.8795, 48.9302) -> (83.164, 49.1637)
  line L1539 (82.5734, 48.7256) -> (82.8795, 48.9302)
  line L1540 (78.4105, 48.9302) -> (78.7166, 48.7256)
  arc A4394 (77.1075, 50.2785) -> (77.4008, 50.4) centre (77.2542, 50.3392) ccw
  arc A4395 (77.7549, 49.8092) -> (77.5094, 49.6078) centre (77.6321, 49.7085) ccw
  arc A4396 (77.5596, 50.1028) -> (77.2956, 49.9264) centre (77.4276, 50.0146) ccw
  arc A4397 (79.4274, 48.5632) -> (79.3352, 48.2593) centre (79.3813, 48.4113) ccw
  arc A4398 (81.9548, 48.2593) -> (81.8626, 48.5632) centre (81.9087, 48.4113) ccw
  arc A4399 (79.3206, 48.2646) -> (79.4421, 48.5579) centre (79.3813, 48.4113) ccw
  arc A4400 (77.2876, 49.9398) -> (77.5676, 50.0894) centre (77.4276, 50.0146) ccw
  line L1541 (80.0946, 48.2326) -> (80.3275, 48.2096)
  line L1542 (80.3275, 48.2096) -> (80.3275, 51.6255)
  arc A4401 (80.3275, 51.7842) -> (80.3275, 51.4667) centre (80.3275, 51.6255) ccw
  arc A4402 (80.3119, 48.0517) -> (80.3431, 48.3676) centre (80.3275, 48.2097) ccw
  arc A4403 (84.0248, 50.7254) -> (84.3287, 50.6332) centre (84.1767, 50.6793) ccw
  line L1543 (68.5509, 3.4741) -> (68.5351, 3.5536)
  line L1544 (83.6578, 49.7085) -> (83.8624, 50.0146)
  arc A4404 (68.4001, 1.0601) -> (68.7176, 1.0601) centre (68.5589, 1.0601) ccw
  arc A4405 (68.5292, 3.9333) -> (68.2652, 3.7569) centre (68.3972, 3.8451) ccw
  arc A4406 (68.3831, 3.5075) -> (68.687, 3.5997) centre (68.535, 3.5536) ccw
  line L1545 (68.5115, 3.6312) -> (68.4805, 3.7062)
  arc A4407 (68.2745, 3.7444) -> (68.5199, 3.9458) centre (68.3972, 3.8451) ccw
  line L1546 (83.164, 49.1637) -> (83.4243, 49.424)
  line L1547 (68.3457, 3.9078) -> (68.2884, 3.9652)
  arc A4408 (83.5258, 49.7967) -> (83.7898, 49.6203) centre (83.6578, 49.7085) ccw
  line L1548 (84.2253, 0.7747) -> (68.4918, 0.7747)
  line L1549 (68.5115, 0.8222) -> (68.5351, 0.8998)
  arc A4409 (68.7066, 0.9484) -> (68.3952, 1.0104) centre (68.5509, 0.9794) ccw
  arc A4410 (84.1759, 50.2644) -> (83.8959, 50.4141) centre (84.0359, 50.3392) ccw
  arc A4411 (68.4918, 0.9334) -> (68.4918, 0.6159) centre (68.4918, 0.7747) ccw
  arc A4412 (84.3772, 50.7933) -> (84.0734, 50.8855) centre (84.2253, 50.8394) ccw
  arc A4413 (68.5822, 3.8525) -> (68.3022, 3.7029) centre (68.4422, 3.7777) ccw
  arc A4414 (68.3405, 3.6313) -> (68.6205, 3.781) centre (68.4805, 3.7062) ccw
  arc A4415 (68.7176, 3.3934) -> (68.4001, 3.3934) centre (68.5589, 3.3934) ccw
  arc A4416 (84.2253, 0.6159) -> (84.2253, 0.9334) centre (84.2253, 0.7747) ccw
  arc A4417 (68.3952, 3.4431) -> (68.7066, 3.505) centre (68.5509, 3.474) ccw
  arc A4418 (84.3234, 50.6186) -> (84.0301, 50.7401) centre (84.1767, 50.6794) ccw
  arc A4419 (83.0518, 49.2759) -> (83.2763, 49.0514) centre (83.1641, 49.1637) ccw
  line L1550 (68.5588, 1.0601) -> (68.5588, 3.3934)
  arc A4420 (83.7223, 50.0894) -> (84.0024, 49.9398) centre (83.8624, 50.0146) ccw
  arc A4421 (68.7089, 3.4896) -> (68.3929, 3.4585) centre (68.5509, 3.474) ccw
  line L1551 (68.5351, 0.8998) -> (68.5509, 0.9794)
  arc A4422 (84.0666, 0.7747) -> (84.3841, 0.7747) centre (84.2253, 0.7747) ccw
  arc A4423 (68.4684, 4.0085) -> (68.223, 3.8071) centre (68.3457, 3.9078) ccw
  line L1552 (83.4243, 49.424) -> (83.6578, 49.7085)
  line L1553 (68.3972, 3.8451) -> (68.3457, 3.9078)
  arc A4424 (68.3452, 0.8355) -> (68.6385, 0.7139) centre (68.4919, 0.7747) ccw
  line L1554 (84.0359, 50.3392) -> (84.1767, 50.6793)
  arc A4425 (68.7168, 1.0446) -> (68.4008, 1.0757) centre (68.5588, 1.0601) ccw
  arc A4426 (83.9943, 49.9264) -> (83.7304, 50.1028) centre (83.8624, 50.0146) ccw
  arc A4427 (68.6634, 3.6773) -> (68.3596, 3.5852) centre (68.5115, 3.6312) ccw
  line L1555 (68.4918, 0.7747) -> (68.5115, 0.8222)
  arc A4428 (68.3596, 0.8683) -> (68.6634, 0.7761) centre (68.5115, 0.8222) ccw
  arc A4429 (68.6271, 3.7669) -> (68.3338, 3.6454) centre (68.4805, 3.7062) ccw
  arc A4430 (68.3929, 0.995) -> (68.7089, 0.9638) centre (68.5509, 0.9794) ccw
  arc A4431 (68.3794, 0.9308) -> (68.6908, 0.8689) centre (68.5351, 0.8999) ccw
  line L1556 (68.5588, 3.3934) -> (68.5509, 3.4741)
  line L1557 (68.4805, 3.7062) -> (68.4422, 3.7777)
  arc A4432 (68.4006, 4.0774) -> (68.1761, 3.8529) centre (68.2884, 3.9651) ccw
  line L1558 (68.5509, 0.9794) -> (68.5588, 1.0601)
  line L1559 (68.5351, 3.5536) -> (68.5115, 3.6312)
  arc A4433 (83.8892, 50.4) -> (84.1825, 50.2785) centre (84.0359, 50.3393) ccw
  arc A4434 (83.7806, 49.6078) -> (83.5351, 49.8092) centre (83.6579, 49.7085) ccw
  arc A4435 (68.3102, 3.6895) -> (68.5742, 3.8659) centre (68.4422, 3.7777) ccw
  arc A4436 (68.6908, 3.5846) -> (68.3794, 3.5227) centre (68.5351, 3.5537) ccw
  arc A4437 (82.7788, 49.0529) -> (82.9802, 48.8074) centre (82.8795, 48.9301) ccw
  arc A4438 (84.3841, 50.8394) -> (84.0666, 50.8394) centre (84.2253, 50.8394) ccw
  arc A4439 (83.5366, 49.3117) -> (83.3121, 49.5362) centre (83.4244, 49.424) ccw
  line L1560 (84.2253, 50.8394) -> (84.2253, 0.7747)
  arc A4440 (68.4008, 3.3778) -> (68.7168, 3.4089) centre (68.5588, 3.3934) ccw
  arc A4441 (68.687, 0.8538) -> (68.3831, 0.9459) centre (68.535, 0.8998) ccw
  line L1561 (83.8624, 50.0146) -> (84.0359, 50.3392)
  arc A4442 (68.3648, 3.5705) -> (68.6582, 3.692) centre (68.5115, 3.6312) ccw
  line L1562 (68.4422, 3.7777) -> (68.3972, 3.8451)
  arc A4443 (68.6582, 0.7615) -> (68.3648, 0.883) centre (68.5115, 0.8222) ccw
  arc A4444 (83.2647, 49.041) -> (83.0633, 49.2864) centre (83.164, 49.1637) ccw
  arc A4445 (33.749, 4.337) -> (33.749, 4.0195) centre (33.749, 4.1783) ccw
  line L1563 (67.8546, 4.1703) -> (67.7739, 4.1783)
  arc A4446 (33.3467, 3.8529) -> (33.1222, 4.0774) centre (33.2345, 3.9652) ccw
  line L1564 (33.1257, 3.8451) -> (33.0806, 3.7777)
  arc A4447 (67.839, 4.0124) -> (67.8702, 4.3283) centre (67.8546, 4.1704) ccw
  arc A4448 (32.8647, 3.692) -> (33.158, 3.5705) centre (33.0114, 3.6312) ccw
  line L1565 (33.0424, 3.7062) -> (33.0113, 3.6312)
  line L1566 (33.749, 4.1783) -> (33.6683, 4.1703)
  arc A4449 (32.9024, 3.781) -> (33.1824, 3.6313) centre (33.0424, 3.7062) ccw
  arc A4450 (32.8359, 3.5997) -> (33.1397, 3.5075) centre (32.9878, 3.5536) ccw
  line L1567 (68.0118, 4.131) -> (67.9342, 4.1545)
  arc A4451 (33.6527, 4.3283) -> (33.6838, 4.0124) centre (33.6683, 4.1704) ccw
  line L1568 (68.2257, 4.0166) -> (68.1582, 4.0617)
  arc A4452 (67.7894, 4.3363) -> (67.7583, 4.0203) centre (67.7739, 4.1783) ccw
  line L1569 (68.1582, 4.0617) -> (68.0867, 4.0999)
  arc A4453 (67.9802, 4.3064) -> (67.8881, 4.0026) centre (67.9341, 4.1545) ccw
  line L1570 (33.4362, 4.0999) -> (33.3646, 4.0617)
  line L1571 (33.0806, 3.7777) -> (33.0424, 3.7062)
  arc A4454 (33.2577, 3.7569) -> (32.9937, 3.9333) centre (33.1257, 3.8451) ccw
  arc A4455 (33.3754, 4.2466) -> (33.4969, 3.9533) centre (33.4361, 4.0999) ccw
  line L1572 (33.3646, 4.0617) -> (33.2972, 4.0166)
  arc A4456 (32.9486, 3.8659) -> (33.2126, 3.6895) centre (33.0806, 3.7777) ccw
  arc A4457 (68.2335, 3.7956) -> (68.458, 4.0201) centre (68.3458, 3.9079) ccw
  arc A4458 (33.3979, 3.8939) -> (33.1965, 4.1394) centre (33.2972, 4.0167) ccw
  arc A4459 (83.3016, 49.5247) -> (83.547, 49.3233) centre (83.4243, 49.424) ccw
  line L1573 (33.1771, 3.9078) -> (33.1257, 3.8451)
  arc A4460 (33.2998, 3.8071) -> (33.0544, 4.0085) centre (33.1771, 3.9078) ccw
  arc A4461 (33.6348, 4.0026) -> (33.5426, 4.3064) centre (33.5887, 4.1545) ccw
  arc A4462 (33.2206, 3.7029) -> (32.9406, 3.8525) centre (33.0806, 3.7777) ccw
  line L1574 (67.9342, 4.1545) -> (67.8546, 4.1703)
  arc A4463 (33.7645, 4.0203) -> (33.7334, 4.3363) centre (33.749, 4.1783) ccw
  arc A4464 (68.1375, 3.8846) -> (68.3139, 4.1486) centre (68.2257, 4.0166) ccw
  arc A4465 (67.7739, 4.0195) -> (67.7739, 4.337) centre (67.7739, 4.1783) ccw
  arc A4466 (68.0834, 3.9217) -> (68.2331, 4.2017) centre (68.1583, 4.0617) ccw
  arc A4467 (33.5718, 3.9843) -> (33.4503, 4.2776) centre (33.5111, 4.131) ccw
  arc A4468 (33.189, 3.6454) -> (32.8957, 3.7669) centre (33.0423, 3.7062) ccw
  arc A4469 (33.2898, 4.2017) -> (33.4395, 3.9217) centre (33.3646, 4.0617) ccw
  arc A4470 (33.511, 3.9599) -> (33.3613, 4.2399) centre (33.4362, 4.0999) ccw
  arc A4471 (33.6992, 4.0146) -> (33.6373, 4.326) centre (33.6683, 4.1703) ccw
  line L1575 (33.5887, 4.1545) -> (33.5111, 4.131)
  arc A4472 (33.209, 4.1486) -> (33.3854, 3.8846) centre (33.2972, 4.0166) ccw
  arc A4473 (68.0725, 4.2776) -> (67.951, 3.9843) centre (68.0118, 4.1309) ccw
  line L1576 (84.1767, 50.6793) -> (84.2253, 50.8394)
  arc A4474 (33.1633, 3.5852) -> (32.8594, 3.6773) centre (33.0114, 3.6312) ccw
  line L1577 (68.2884, 3.9652) -> (68.2257, 4.0166)
  arc A4475 (68.1615, 4.2399) -> (68.0119, 3.9599) centre (68.0867, 4.0999) ccw
  line L1578 (67.7739, 4.1783) -> (33.749, 4.1783)
  arc A4476 (67.9657, 3.9791) -> (68.0579, 4.2829) centre (68.0118, 4.131) ccw
  line L1579 (33.0113, 3.6312) -> (32.9878, 3.5536)
  arc A4477 (67.9032, 3.9988) -> (67.9651, 4.3102) centre (67.9342, 4.1545) ccw
  arc A4478 (33.465, 4.2829) -> (33.5572, 3.9791) centre (33.5111, 4.131) ccw
  arc A4479 (33.1338, 4.0879) -> (33.3352, 3.8425) centre (33.2345, 3.9652) ccw
  arc A4480 (33.4528, 3.9297) -> (33.2764, 4.1937) centre (33.3646, 4.0617) ccw
  arc A4481 (68.1877, 3.8425) -> (68.3891, 4.0879) centre (68.2884, 3.9652) ccw
  line L1580 (33.6683, 4.1703) -> (33.5887, 4.1545)
  line L1581 (33.2972, 4.0166) -> (33.2345, 3.9652)
  arc A4482 (68.3264, 4.1394) -> (68.125, 3.8939) centre (68.2257, 4.0166) ccw
  arc A4483 (33.0649, 4.0201) -> (33.2894, 3.7956) centre (33.1772, 3.9079) ccw
  line L1582 (33.2345, 3.9652) -> (33.1771, 3.9078)
  arc A4484 (68.026, 3.9533) -> (68.1475, 4.2466) centre (68.0867, 4.1) ccw
  arc A4485 (33.5577, 4.3102) -> (33.6197, 3.9988) centre (33.5887, 4.1545) ccw
  arc A4486 (1.1732, 49.6203) -> (1.4371, 49.7967) centre (1.3051, 49.7085) ccw
  line L1583 (0.7863, 50.6793) -> (0.9271, 50.3392)
  arc A4487 (0.9266, 50.7635) -> (0.6228, 50.6713) centre (0.7747, 50.7174) ccw
  arc A4488 (33.122, 1.0757) -> (32.806, 1.0446) centre (32.964, 1.0601) ccw
  line L1584 (32.964, 1.0601) -> (32.972, 0.9794)
  arc A4489 (0.9329, 50.7401) -> (0.6396, 50.6186) centre (0.7863, 50.6793) ccw
  arc A4490 (32.814, 0.9638) -> (33.13, 0.995) centre (32.972, 0.9794) ccw
  arc A4491 (32.806, 3.4089) -> (33.122, 3.3778) centre (32.964, 3.3933) ccw
  line L1585 (3.0543, 48.4113) -> (3.4066, 48.3044)
  line L1586 (1.1006, 50.0146) -> (1.3052, 49.7085)
  arc A4492 (1.6867, 49.0514) -> (1.9112, 49.2759) centre (1.799, 49.1637) ccw
  arc A4493 (32.8844, 0.7139) -> (33.1777, 0.8355) centre (33.0311, 0.7747) ccw
  arc A4494 (3.3605, 48.1525) -> (3.4527, 48.4563) centre (3.4066, 48.3044) ccw
  arc A4495 (33.13, 3.4585) -> (32.814, 3.4896) centre (32.972, 3.4741) ccw
  line L1587 (2.0835, 48.9302) -> (2.3896, 48.7256)
  line L1588 (1.5387, 49.424) -> (1.799, 49.1637)
  arc A4496 (1.8997, 49.2864) -> (1.6983, 49.041) centre (1.799, 49.1637) ccw
  arc A4497 (3.4375, 48.4601) -> (3.3756, 48.1487) centre (3.4065, 48.3044) ccw
  line L1589 (0.7747, 0.7747) -> (0.7747, 50.7174)
  arc A4498 (32.8321, 0.8689) -> (33.1435, 0.9308) centre (32.9878, 0.8998) ccw
  arc A4499 (33.031, 0.6159) -> (33.031, 0.9334) centre (33.031, 0.7747) ccw
  arc A4500 (1.2326, 50.1028) -> (0.9686, 49.9264) centre (1.1006, 50.0146) ccw
  arc A4501 (32.8594, 0.7761) -> (33.1633, 0.8683) centre (33.0114, 0.8222) ccw
  arc A4502 (68.2464, 4.1937) -> (68.07, 3.9297) centre (68.1582, 4.0617) ccw
  arc A4503 (33.003, 3.9458) -> (33.2484, 3.7444) centre (33.1257, 3.8451) ccw
  arc A4504 (33.158, 0.883) -> (32.8647, 0.7615) centre (33.0114, 0.8222) ccw
  arc A4505 (33.1397, 0.9459) -> (32.8359, 0.8538) centre (32.9878, 0.8999) ccw
  line L1590 (3.4066, 48.3044) -> (3.7676, 48.2326)
  arc A4506 (1.416, 49.3233) -> (1.6614, 49.5247) centre (1.5387, 49.424) ccw
  arc A4507 (1.9828, 48.8074) -> (2.1842, 49.0529) centre (2.0835, 48.9301) ccw
  arc A4508 (0.7805, 50.2785) -> (1.0738, 50.4) centre (0.9272, 50.3392) ccw
  line L1591 (2.3896, 48.7256) -> (2.7142, 48.5521)
  line L1592 (32.9878, 0.8998) -> (33.0113, 0.8222)
  arc A4509 (1.6509, 49.5362) -> (1.4264, 49.3117) centre (1.5387, 49.424) ccw
  arc A4510 (2.6394, 48.4121) -> (2.7891, 48.6921) centre (2.7143, 48.5521) ccw
  line L1593 (33.5111, 4.131) -> (33.4362, 4.0999)
  arc A4511 (3.7366, 48.0769) -> (3.7986, 48.3883) centre (3.7676, 48.2326) ccw
  arc A4512 (2.4644, 48.8656) -> (2.3148, 48.5856) centre (2.3896, 48.7256) ccw
  arc A4513 (33.1435, 3.5227) -> (32.8321, 3.5846) centre (32.9878, 3.5537) ccw
  line L1594 (1.799, 49.1637) -> (2.0835, 48.9302)
  arc A4514 (33.1277, 1.0104) -> (32.8163, 0.9484) centre (32.972, 0.9794) ccw
  line L1595 (2.7142, 48.5521) -> (3.0543, 48.4113)
  line L1596 (68.0867, 4.0999) -> (68.0118, 4.131)
  arc A4515 (1.4279, 49.8092) -> (1.1824, 49.6078) centre (1.3051, 49.7085) ccw
  arc A4516 (2.1717, 49.0621) -> (1.9953, 48.7982) centre (2.0835, 48.9302) ccw
  line L1597 (33.0113, 0.8222) -> (33.031, 0.7747)
  arc A4517 (32.8163, 3.505) -> (33.1277, 3.4431) centre (32.972, 3.474) ccw
  arc A4518 (32.8053, 1.0601) -> (33.1228, 1.0601) centre (32.9641, 1.0601) ccw
  line L1598 (33.031, 0.7747) -> (0.7747, 0.7747)
  arc A4519 (3.1004, 48.5632) -> (3.0082, 48.2593) centre (3.0543, 48.4113) ccw
  arc A4520 (2.3014, 48.5936) -> (2.4778, 48.8576) centre (2.3896, 48.7256) ccw
  arc A4521 (0.9334, 50.7174) -> (0.6159, 50.7174) centre (0.7747, 50.7174) ccw
  arc A4522 (67.8856, 4.326) -> (67.8236, 4.0146) centre (67.8546, 4.1703) ccw
  line L1599 (0.9271, 50.3392) -> (1.1006, 50.0146)
  arc A4523 (0.6343, 50.6332) -> (0.9382, 50.7254) centre (0.7863, 50.6793) ccw
  line L1600 (1.3052, 49.7085) -> (1.5387, 49.424)
  arc A4524 (2.9936, 48.2646) -> (3.1151, 48.5579) centre (3.0543, 48.4112) ccw
  arc A4525 (0.9606, 49.9398) -> (1.2406, 50.0894) centre (1.1006, 50.0146) ccw
  line L1601 (3.7676, 48.2326) -> (4.0005, 48.2096)
  arc A4526 (0.6159, 0.7747) -> (0.9334, 0.7747) centre (0.7747, 0.7747) ccw
  arc A4527 (33.1228, 3.3934) -> (32.8053, 3.3934) centre (32.9641, 3.3934) ccw
  arc A4528 (8.1085, 50.9855) -> (7.8047, 51.0777) centre (7.9566, 51.0316) ccw
  arc A4529 (8.0514, 52.1017) -> (8.0514, 52.4192) centre (8.0514, 52.2604) ccw
  arc A4530 (4.6199, 48.3676) -> (4.6511, 48.0517) centre (4.6355, 48.2097) ccw
  arc A4531 (3.9849, 48.0517) -> (4.0161, 48.3676) centre (4.0005, 48.2097) ccw
  arc A4532 (4.4768, 51.6255) -> (4.7943, 51.6255) centre (4.6356, 51.6255) ccw
  line L1602 (0.7747, 50.7174) -> (0.7863, 50.6793)
  arc A4533 (7.2096, 49.3117) -> (6.9851, 49.5362) centre (7.0974, 49.424) ccw
  arc A4534 (4.1593, 51.6255) -> (3.8418, 51.6255) centre (4.0005, 51.6255) ccw
  arc A4535 (4.4767, 48.2096) -> (4.7942, 48.2096) centre (4.6355, 48.2096) ccw
  arc A4536 (5.6278, 48.2593) -> (5.5356, 48.5632) centre (5.5817, 48.4113) ccw
  line L1603 (4.6355, 48.2096) -> (4.8684, 48.2326)
  line L1604 (4.0005, 48.2096) -> (4.0005, 51.6255)
  arc A4537 (1.0671, 50.4141) -> (0.7871, 50.2644) centre (0.9271, 50.3392) ccw
  arc A4538 (4.8839, 48.0746) -> (4.8528, 48.3906) centre (4.8683, 48.2326) ccw
  arc A4539 (7.3953, 50.0894) -> (7.6754, 49.9398) centre (7.5353, 50.0146) ccw
  arc A4540 (4.6355, 51.7843) -> (4.6355, 51.4668) centre (4.6355, 51.6256) ccw
  line L1605 (4.6355, 51.6255) -> (4.6355, 52.2605)
  line L1606 (7.9566, 51.0316) -> (8.0284, 51.3926)
  arc A4541 (7.9964, 50.6186) -> (7.7031, 50.7401) centre (7.8498, 50.6793) ccw
  arc A4542 (4.0005, 51.7842) -> (4.0005, 51.4667) centre (4.0005, 51.6255) ccw
  arc A4543 (3.7832, 48.3906) -> (3.752, 48.0746) centre (3.7676, 48.2326) ccw
  line L1607 (5.5817, 48.4113) -> (5.9218, 48.5521)
  arc A4544 (4.7943, 52.2605) -> (4.4768, 52.2605) centre (4.6356, 52.2605) ccw
  line L1608 (4.6355, 52.2605) -> (8.0514, 52.2605)
  arc A4545 (4.6355, 51.4667) -> (4.6355, 51.7842) centre (4.6355, 51.6255) ccw
  line L1609 (4.0005, 51.6255) -> (4.6355, 51.6255)
  line L1610 (32.972, 0.9794) -> (32.9878, 0.8998)
  arc A4546 (6.3212, 48.5856) -> (6.1716, 48.8656) centre (6.2464, 48.7256) ccw
  line L1611 (6.2464, 48.7256) -> (6.5525, 48.9302)
  arc A4547 (6.9746, 49.5247) -> (7.22, 49.3233) centre (7.0973, 49.424) ccw
  arc A4548 (5.8469, 48.6921) -> (5.9966, 48.4121) centre (5.9218, 48.5521) ccw
  arc A4549 (8.2093, 51.6099) -> (7.8934, 51.6411) centre (8.0513, 51.6255) ccw
  arc A4550 (6.4518, 49.0529) -> (6.6532, 48.8074) centre (6.5525, 48.9301) ccw
  line L1612 (32.964, 3.3934) -> (32.964, 1.0601)
  arc A4551 (7.8704, 51.4082) -> (8.1864, 51.377) centre (8.0284, 51.3926) ccw
  arc A4552 (3.8418, 48.2096) -> (4.1593, 48.2096) centre (4.0005, 48.2096) ccw
  line L1613 (7.8497, 50.6793) -> (7.9566, 51.0316)
  line L1614 (7.3308, 49.7085) -> (7.5354, 50.0146)
  arc A4553 (5.5209, 48.5579) -> (5.6424, 48.2646) centre (5.5816, 48.4112) ccw
  arc A4554 (8.1841, 51.3616) -> (7.8727, 51.4236) centre (8.0284, 51.3926) ccw
  arc A4555 (4.8374, 48.3883) -> (4.8994, 48.0769) centre (4.8684, 48.2326) ccw
  arc A4556 (7.8009, 51.0625) -> (8.1123, 51.0006) centre (7.9566, 51.0316) ccw
  line L1615 (5.2294, 48.3044) -> (5.5817, 48.4113)
  arc A4557 (7.8489, 50.2644) -> (7.5689, 50.4141) centre (7.7089, 50.3392) ccw
  arc A4558 (0.7747, 0.9334) -> (0.7747, 0.6159) centre (0.7747, 0.7747) ccw
  arc A4559 (7.6978, 50.7254) -> (8.0017, 50.6332) centre (7.8498, 50.6793) ccw
  line L1616 (32.9878, 3.5536) -> (32.972, 3.4741)
  line L1617 (7.5354, 50.0146) -> (7.7089, 50.3392)
  arc A4560 (8.0514, 51.4668) -> (8.0514, 51.7843) centre (8.0514, 51.6256) ccw
  line L1618 (32.972, 3.4741) -> (32.964, 3.3934)
  line L1619 (5.9218, 48.5521) -> (6.2464, 48.7256)
  line L1620 (8.0284, 51.3926) -> (8.0514, 51.6255)
  line L1621 (8.0514, 51.6255) -> (4.6355, 51.6255)
  arc A4561 (6.7248, 49.2759) -> (6.9493, 49.0514) centre (6.8371, 49.1637) ccw
  line L1622 (4.8684, 48.2326) -> (5.2294, 48.3044)
  arc A4562 (5.1833, 48.4563) -> (5.2755, 48.1525) centre (5.2294, 48.3044) ccw
  arc A4563 (2.775, 48.6988) -> (2.6535, 48.4055) centre (2.7143, 48.5522) ccw
  arc A4564 (5.2604, 48.1487) -> (5.1985, 48.4601) centre (5.2294, 48.3044) ccw
  line L1623 (6.837, 49.1637) -> (7.0973, 49.424)
  arc A4565 (4.7942, 51.6255) -> (4.4767, 51.6255) centre (4.6355, 51.6255) ccw
  line L1624 (7.0973, 49.424) -> (7.3308, 49.7085)
  arc A4566 (7.6673, 49.9264) -> (7.4034, 50.1028) centre (7.5353, 50.0146) ccw
  arc A4567 (71.3694, 40.4649) -> (71.3694, 40.7824) centre (71.3694, 40.6237) ccw
  line L1625 (70.4098, 40.4328) -> (70.3249, 40.3479)
  arc A4568 (7.4536, 49.6078) -> (7.2081, 49.8092) centre (7.3309, 49.7085) ccw
  arc A4569 (5.4611, 55.6772) -> (5.3689, 55.3734) centre (5.415, 55.5253) ccw
  arc A4570 (6.4643, 54.8238) -> (6.6407, 55.0878) centre (6.5525, 54.9558) ccw
  arc A4571 (72.227, 39.5586) -> (72.5204, 39.6801) centre (72.3737, 39.6194) ccw
  arc A4572 (70.3491, 40.5795) -> (70.4706, 40.2862) centre (70.4099, 40.4329) ccw
  arc A4573 (7.6754, 53.9462) -> (7.3953, 53.7966) centre (7.5353, 53.8714) ccw
  arc A4574 (6.6532, 55.0786) -> (6.4518, 54.8331) centre (6.5525, 54.9558) ccw
  line L1626 (6.837, 54.7223) -> (6.5525, 54.9558)